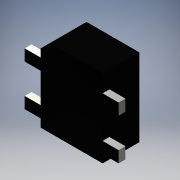
# Autodesk Inventor part: QRE1113GR
Saved by Autodesk Inventor 2016 (Build 200138000, 138)
## iProperties
Created: 2016-01-30
Part Number: QRE1113GR
Material: Generic
Document SubType Name: Modeling
Designer: jferner
Density: 1 g/cm^3
Appearance: Default
QRE1113GR_z: 1.600 mm
QRE1113GR_x: 2.700 mm
QRE1113GR_y: 3.400 mm
Author: jferner
Autodesk Inventor part; units mm, degrees
ref_plane "YZ Plane" through (0, 0, 0) normal (1, 0, 0) x (0, 1, 0)
ref_plane "XZ Plane" through (0, 0, 0) normal (0, 1, 0) x (-1, 0, 0)
ref_plane "XY Plane" through (0, 0, 0) normal (0, 0, 1) x (1, 0, 0)
sketch "Sketch1" plane through (0, 0, 0) normal (0, 1, 0) x (-1, 0, 0)
  line L0 (0, 0) -> (-2.7, 0)
  line L1 (-2.7, 0) -> (-2.7, 3.4)
  line L2 (-2.7, 3.4) -> (-0.4, 3.4)
  line L3 (0, 3) -> (0, 0)
  line L4 (0, 3) -> (-0.4, 3.4)
  dimension "QRE1113GR_x" = 2.7
  dimension "QRE1113GR_y" = 3.4
  dimension "d2" = 45
  dimension "d3" = 2.3
  constraints: 10 end point, 2 parallel, 1 horizontal, 1 perpendicular
  measures "QRE1113GR_x" distance of L0.start L0.end
  measures "QRE1113GR_y" distance of L0.end L1.end
  measures "d2" angle of L2 L4
  measures "d3" distance of L2.end L1.end
extrude "Extrusion1" add sketch "Sketch1" along normal blind 1.6
sketch "Sketch2" plane through (0, 0, 0) normal (-1, 0, 0) x (0, 0, 1)
  line L0 (3, 0) -> (0, 0) projected
  line L1 (0.35, 0) -> (0.85, 0)
  line L2 (0.85, 0) -> (0.85, 0.3)
  line L3 (0.85, 0.3) -> (0.35, 0.3)
  line L4 (0.35, 0.3) -> (0.35, 0)
  line L5 (2.15, 0) -> (2.65, 0)
  line L6 (0, 1.6) -> (3, 1.6) projected
  line L7 (1.5, 1.6) -> (1.5, 0)
  line L8 (0.6, 0.3) -> (0.6, 0)
  dimension "d6" = 0.5
  dimension "d7" = 0.3
  dimension "d8" = 0.9
  constraints: 14 end point, 3 midpoint, 3 point on line, 2 horizontal, 2 parallel, 2 perpendicular
  measures "d6" distance of L2.end L3.end
  measures "d7" distance of L3.end L1.start
  measures "d8" distance between parallel lines of L7 L8
extrude "Extrusion2" add sketch "Sketch2" along normal blind 0.7
pattern_linear "Rectangular Pattern1" count 2 spacing 1.8 along (0, 0, 1) count 2 spacing 3.4 along (1, 0, 0) of "Extrusion2"
body "Solid1"
